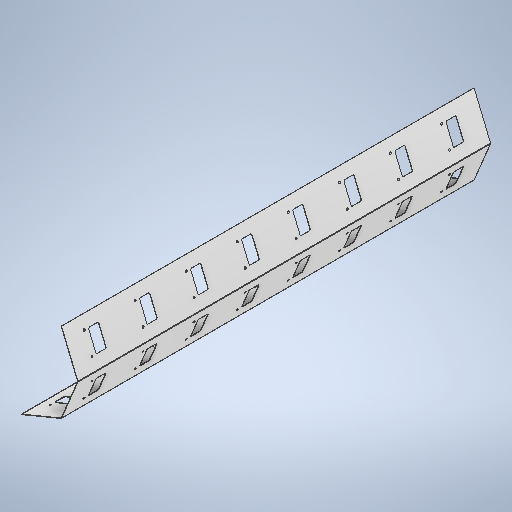
# Autodesk Inventor part: DMF 01 14 Барабан Лист прав брт v2.1
Saved by Autodesk Inventor 2025 (Build 290162010, 162A)
## iProperties
Created: 2024-04-28
Part Number: DMF 01 14 Барабан Лист прав брт v2.1
Material: Stainless Steel AISI 304
Document SubType Name: Sheet Metal
Designer: pokla
Density: 8 g/cm^3
Appearance: Chrome - Satin
Sheet Metal Rule: Default
Flat Pattern Width: 63.3571 cm
Flat Pattern Length: 202 cm
Flat Pattern Area: 12798.1 cm^2
Sheet Metal Width: 633,571 mm
Sheet Metal Length: 2020,000 mm
Sheet Metal Area: 1279813,721 mm^2
Stock Number: Барабан_Лист_Правый_Борт
Author: pokla
Autodesk Inventor part; units mm, degrees
ref_plane "YZ Plane" through (0, 0, 0) normal (1, 0, 0) x (0, 1, 0)
ref_plane "XZ Plane" through (0, 0, 0) normal (0, 1, 0) x (-1, 0, 0)
ref_plane "XY Plane" through (0, 0, 0) normal (0, 0, 1) x (1, 0, 0)
sketch "Sketch2" plane through (0, 0, 0) normal (0, 0, 1) x (1, 0, 0)
  line L0 (0, 277.633599) -> (196.316601, 196.316601) construction
  line L1 (196.316601, 196.316601) -> (277.633599, 0) construction
  line L2 (277.633599, 0) -> (196.316601, -196.316601) construction
  line L3 (196.316601, -196.316601) -> (0, -277.633599) construction
  line L4 (0, -277.633599) -> (-196.316601, -196.316601) construction
  line L5 (-196.316601, -196.316601) -> (-277.633599, 0) construction
  line L6 (-277.633599, 0) -> (-196.316601, 196.316601) construction
  line L7 (-196.316601, 196.316601) -> (0, 277.633599) construction
  line L8 (196.661016, 195.485109) -> (276.999549, 1.530734)
  line L9 (276.999549, -1.530734) -> (196.950651, -194.785867)
  arc A0 (276.999549, -1.530734) -> (276.999549, 1.530734) centre (273.304031, 0) ccw
  line L10 (194.785867, -196.950651) -> (0.831492, -277.289184)
  arc A1 (194.785867, -196.950651) -> (196.950651, -194.785867) centre (193.255133, -193.255133) ccw
  line L11 (277.633599, 0) -> (276.999549, 1.530734) construction
  line L12 (276.999549, 1.530734) -> (278.530282, 2.164784) construction
  line L13 (278.530282, 2.164784) -> (279.164333, 0.634051) construction
  line L14 (279.164333, 0.634051) -> (277.633599, 0) construction
  line L15 (1.530734, 276.999549) -> (0, 277.633599) construction
  line L16 (0, 277.633599) -> (0.634051, 279.164333) construction
  line L17 (0.634051, 279.164333) -> (2.164784, 278.530282) construction
  line L18 (2.164784, 278.530282) -> (1.530734, 276.999549) construction
  point P0 (0, 0)
  point P1 (0, 0)
  dimension "d56" = 513
  dimension "d58" = 4
  dimension "d69" = 0.9
  dimension "d70" = 4
  dimension "d149" = 0.9
  measures "d56" distance between parallel lines of L6 L2
  measures "d58" radius of A0
  measures "d69" distance of L3.end L10.end
  measures "d70" radius of A1
  measures "d149" distance of L0.end L8.start
contour flange "Contour Flange2" sketch "Sketch2" thickness 2 bend radius 2 width 2020 along (0, 0, 1) mid plane no both sides no wall seen from (236.830282, 98.507921, 0) lies toward (-0.9238795, -0.3826834, 0) curves L8 A0 L9 A1 L10
bend "Bend2"
corner "Corner2"
sketch "Sketch13" plane through (196.950651, -194.785867, 2020) normal (0.9238795, -0.3826834, 0) x (0, 0, -1)
  line L0 (110, 154.588924) -> (160, 154.588924)
  line L1 (160, 154.588924) -> (160, 54.588924)
  line L2 (160, 54.588924) -> (110, 54.588924)
  line L3 (110, 54.588924) -> (110, 154.588924)
  circle A0 centre (90, 154.588924) radius 4.5
  circle A1 centre (90, 54.588924) radius 4.5
  line L4 (160, 104.588924) -> (110, 104.588924) construction
  line L5 (0, 0) -> (0, 209.177849)
  point P0 (2020, 104.588924)
  point P1 (0, 104.588924)
  dimension "d150" = 9
  dimension "d151" = 100
  dimension "d152" = 50
  dimension "d153" = 20
  dimension "d154" = 100
  dimension "d155" = 110
  constraints: 10 end point, 3 midpoint, 2 centre point, 2 parallel, 1 horizontal, 1 horizontal alignment, 1 perpendicular, 1 other
  measures "d150" diameter of A0
  measures "d151" distance of L2.end L0.start
  measures "d152" distance of L0.start L0.end
  measures "d153" distance from line of A0.centre L3
  measures "d154" distance of A1.centre A0.centre
  measures "d155" distance between parallel lines of L5 L3
extrude "Cut2" cut sketch "Sketch13" against normal blind 2
fillet "Fillet3" radius 5 4 edges at (255.1854, -51.5816, 1860) (255.1854, -51.5816, 1910) (216.917, -143.9696, 1910) (216.917, -143.9696, 1860)
pattern_linear "Rectangular Pattern4" count 8 spacing 250 along (0, 0, -1) of "Cut2", "Fillet3"
pattern_circular "Circular Pattern3" count 3 over 90 about axis through (0, 0, -10) along (0, 0, 1) of "Cut2", "Fillet3", "Rectangular Pattern4" both ways yes
equation "\"d56\" = Барабан_габарит_по_кассетам"
equation "\"d58\" = BendRadius + Thickness"
equation "\"d69\" = Барабан_отступ_развертки"
equation "\"d70\" = BendRadius + Thickness"
equation "\"d25\" = Thickness"
equation "\"d26\" = BendReliefWidth"
equation "\"d27\" = BendReliefDepth"
equation "\"d28\" = MinimumRemnant"
equation "\"d29\" = TransitionRadius"
equation "\"d31\" = BendRadius"
equation "\"d33\" = CornerReliefSize"
equation "\"d34\" = GapSize"
equation "\"d35\" = JacobiRadiusSize"
equation "\"BendRadius\" = Thickness"
equation "\"BendReliefWidth\" = Thickness"
equation "\"BendReliefDepth\" = 0.5 * Thickness"
equation "\"CornerReliefSize\" = 4 * Thickness"
equation "\"MinimumRemnant\" = 2 * Thickness"
equation "\"TransitionRadius\" = BendRadius"
equation "\"JacobiRadiusSize\" = BendRadius"
equation "\"GapSize\" = Thickness"
equation "\"Барабан_габарит_по_кассетам\" = 513"
equation "\"Thickness\" = 2"
equation "\"Барабан_отступ_развертки\" = 0.9"
body "Solid2"
